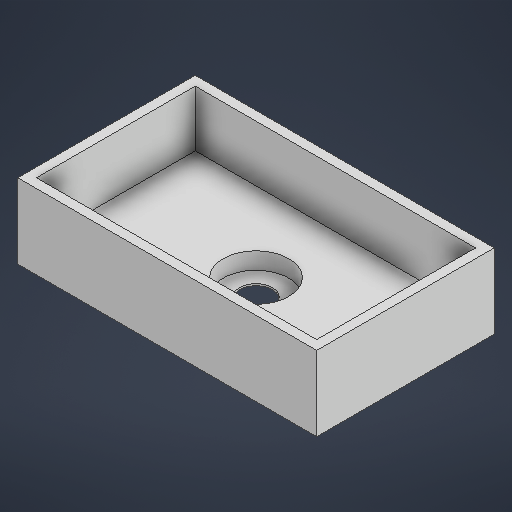
# Autodesk Inventor part: Battery_box
Saved by Autodesk Inventor 2027 (Build 310192060, 192F)
## iProperties
Created: 2026-06-27
Part Number: Battery_box
Material: Ogólny
Document SubType Name: Modeling
Designer: User
Density: 1 g/cm^3
Appearance: Domyślna
Author: User
Autodesk Inventor part; units mm, degrees
ref_plane "YZ Plane" through (0, 0, 0) normal (1, 0, 0) x (0, 1, 0)
ref_plane "XZ Plane" through (0, 0, 0) normal (0, 1, 0) x (-1, 0, 0)
ref_plane "XY Plane" through (0, 0, 0) normal (0, 0, 1) x (1, 0, 0)
sketch "Szkic1" plane through (0, 0, 0) normal (0, 1, 0) x (-1, 0, 0)
  line L0 (-15, 8.5) -> (15, 8.5)
  line L1 (15, 8.5) -> (15, -8.5)
  line L2 (15, -8.5) -> (-15, -8.5)
  line L3 (-15, -8.5) -> (-15, 8.5)
  line L4 (-15, 8.5) -> (15, -8.5) construction
  line L5 (15, 8.5) -> (-15, -8.5) construction
  line L6 (-16, 9.5) -> (16, 9.5)
  line L7 (16, 9.5) -> (16, -9.5)
  line L8 (16, -9.5) -> (-16, -9.5)
  line L9 (-16, -9.5) -> (-16, 9.5)
  line L10 (-16, 9.5) -> (16, -9.5) construction
  line L11 (16, 9.5) -> (-16, -9.5) construction
  circle A0 centre (0, 0) radius 1.75
  circle A1 centre (0, 0) radius 3.5
  dimension "d0" = 30
  dimension "d1" = 17
  dimension "d2" = 32
  dimension "d3" = 19
  dimension "d4" = 3.5
  dimension "d5" = 7
  constraints: 24 end point, 4 midpoint, 4 parallel, 2 centre point, 2 coincident, 2 horizontal, 2 perpendicular
  measures "d0" distance of L1.end L2.end
  measures "d1" distance of L0.end L1.end
  measures "d2" distance of L7.end L8.end
  measures "d3" distance of L6.end L7.end
  measures "d4" diameter of A0
  measures "d5" diameter of A1
extrude "Wyciągnięcie proste1" add sketch "Szkic1" along normal blind 6 contours L6 L7 L8 L9
extrude "Wyciągnięcie proste2" add sketch "Szkic1" against normal blind 2 contours L0 L1 L2 L3 | L6 L7 L8 L9 | A1
extrude "Wyciągnięcie proste3" cut sketch "Szkic1" against normal blind 1.8 contours A1
